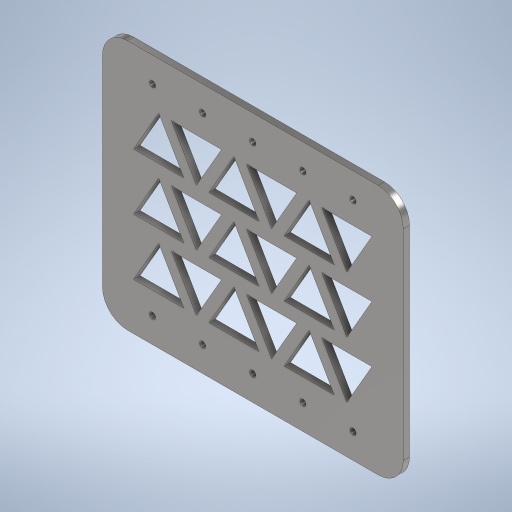
# Autodesk Inventor part: Low Frame to Mid Frame bracket
Saved by Autodesk Inventor 2023 (Build 270158030, 158C)
## iProperties
Created: 2022-07-20
Part Number: Low Frame to Mid Frame bracket
Material: Generic
Document SubType Name: Modeling
Designer: rm0990889
Density: 1 g/cm^3
Appearance: Semi-Polished
Author: rm0990889
Autodesk Inventor part; units mm, degrees
ref_plane "YZ Plane" through (0, 0, 0) normal (1, 0, 0) x (0, 1, 0)
ref_plane "XZ Plane" through (0, 0, 0) normal (0, 1, 0) x (-1, 0, 0)
ref_plane "XY Plane" through (0, 0, 0) normal (0, 0, 1) x (1, 0, 0)
sketch "Sketch1" plane through (0, 0, 0) normal (0, 0, 1) x (1, 0, 0)
  line L0 (0, 0) -> (152.4, 0)
  line L1 (152.4, 25.4) -> (152.4, 127)
  line L2 (152.4, 152.4) -> (0, 152.4)
  line L3 (0, 127) -> (0, 25.4)
  circle A0 centre (25.4, 127) radius 1.5875
  circle A1 centre (50.8, 127) radius 1.5875
  circle A2 centre (76.2, 127) radius 1.5875
  circle A3 centre (101.6, 127) radius 1.5875
  circle A4 centre (127, 127) radius 1.5875
  circle A5 centre (25.4, 25.4) radius 1.5875
  circle A6 centre (50.8, 25.4) radius 1.5875
  circle A7 centre (76.2, 25.4) radius 1.5875
  circle A8 centre (101.6, 25.4) radius 1.5875
  circle A9 centre (127, 25.4) radius 1.5875
  line L4 (41.275, 36.6265) -> (15.875, 36.6265)
  line L5 (15.875, 36.6265) -> (28.575, 58.6235)
  line L6 (28.575, 58.6235) -> (41.275, 36.6265)
  line L7 (60.325, 58.6235) -> (47.625, 36.6265)
  line L8 (47.625, 36.6265) -> (34.925, 58.6235)
  line L9 (34.925, 58.6235) -> (60.325, 58.6235)
  line L10 (98.425, 58.6235) -> (85.725, 36.6265)
  line L11 (73.025, 58.6235) -> (98.425, 58.6235)
  line L12 (85.725, 36.6265) -> (73.025, 58.6235)
  line L13 (66.675, 58.6235) -> (79.375, 36.6265)
  line L14 (53.975, 36.6265) -> (66.675, 58.6235)
  line L15 (79.375, 36.6265) -> (53.975, 36.6265)
  line L16 (136.525, 58.6235) -> (123.825, 36.6265)
  line L17 (111.125, 58.6235) -> (136.525, 58.6235)
  line L18 (123.825, 36.6265) -> (111.125, 58.6235)
  line L19 (104.775, 58.6235) -> (117.475, 36.6265)
  line L20 (92.075, 36.6265) -> (104.775, 58.6235)
  line L21 (117.475, 36.6265) -> (92.075, 36.6265)
  line L22 (0, 36.6265) -> (15.875, 36.6265)
  line L23 (136.525, 58.6235) -> (152.4, 58.6235)
  line L24 (104.775, 87.1985) -> (117.475, 65.2015)
  line L25 (123.825, 65.2015) -> (111.125, 87.1985)
  line L26 (136.525, 87.1985) -> (123.825, 65.2015)
  line L27 (111.125, 87.1985) -> (136.525, 87.1985)
  line L28 (117.475, 65.2015) -> (92.075, 65.2015)
  line L29 (41.275, 65.2015) -> (15.875, 65.2015)
  line L30 (15.875, 65.2015) -> (28.575, 87.1985)
  line L31 (28.575, 87.1985) -> (41.275, 65.2015)
  line L32 (60.325, 87.1985) -> (47.625, 65.2015)
  line L33 (47.625, 65.2015) -> (34.925, 87.1985)
  line L34 (34.925, 87.1985) -> (60.325, 87.1985)
  line L35 (92.075, 65.2015) -> (104.775, 87.1985)
  line L36 (73.025, 87.1985) -> (98.425, 87.1985)
  line L37 (85.725, 65.2015) -> (73.025, 87.1985)
  line L38 (66.675, 87.1985) -> (79.375, 65.2015)
  line L39 (53.975, 65.2015) -> (66.675, 87.1985)
  line L40 (79.375, 65.2015) -> (53.975, 65.2015)
  line L41 (98.425, 87.1985) -> (85.725, 65.2015)
  line L42 (104.775, 115.7735) -> (117.475, 93.7765)
  line L43 (123.825, 93.7765) -> (111.125, 115.7735)
  line L44 (136.525, 115.7735) -> (123.825, 93.7765)
  line L45 (111.125, 115.7735) -> (136.525, 115.7735)
  line L46 (117.475, 93.7765) -> (92.075, 93.7765)
  line L47 (41.275, 93.7765) -> (15.875, 93.7765)
  line L48 (15.875, 93.7765) -> (28.575, 115.7735)
  line L49 (28.575, 115.7735) -> (41.275, 93.7765)
  line L50 (60.325, 115.7735) -> (47.625, 93.7765)
  line L51 (47.625, 93.7765) -> (34.925, 115.7735)
  line L52 (34.925, 115.7735) -> (60.325, 115.7735)
  line L53 (92.075, 93.7765) -> (104.775, 115.7735)
  line L54 (73.025, 115.7735) -> (98.425, 115.7735)
  line L55 (85.725, 93.7765) -> (73.025, 115.7735)
  line L56 (66.675, 115.7735) -> (79.375, 93.7765)
  line L57 (53.975, 93.7765) -> (66.675, 115.7735)
  line L58 (79.375, 93.7765) -> (53.975, 93.7765)
  line L59 (98.425, 115.7735) -> (85.725, 93.7765)
  line L60 (15.875, 36.6265) -> (15.875, 0)
  line L61 (28.575, 115.7735) -> (28.575, 152.4)
  line L62 (12.7, 12.7) -> (139.7, 12.7)
  line L63 (12.7, 139.7) -> (139.7, 139.7)
  arc A10 (0, 25.4) -> (12.7, 12.7) centre (12.7, 25.4) ccw
  arc A11 (139.7, 12.7) -> (152.4, 25.4) centre (139.7, 25.4) ccw
  arc A12 (152.4, 127) -> (139.7, 139.7) centre (139.7, 127) ccw
  arc A13 (12.7, 139.7) -> (0, 127) centre (12.7, 127) ccw
  point P0 (28.575, 43.9588)
  point P1 (28.575, 36.6265)
  point P2 (47.625, 51.2912)
  point P3 (85.725, 51.2912)
  point P4 (66.675, 43.9588)
  point P5 (66.675, 36.6265)
  point P6 (123.825, 51.2912)
  point P7 (104.775, 43.9588)
  point P8 (104.775, 36.6265)
  point P9 (123.825, 79.8662)
  point P10 (104.775, 65.2015)
  point P11 (28.575, 72.5338)
  point P12 (28.575, 65.2015)
  point P13 (47.625, 79.8662)
  point P14 (104.775, 72.5338)
  point P15 (85.725, 79.8662)
  point P16 (66.675, 72.5338)
  point P17 (66.675, 65.2015)
  point P18 (123.825, 108.4412)
  point P19 (104.775, 93.7765)
  point P20 (28.575, 101.1088)
  point P21 (28.575, 93.7765)
  point P22 (47.625, 108.4412)
  point P23 (104.775, 101.1088)
  point P24 (85.725, 108.4412)
  point P25 (66.675, 101.1088)
  point P26 (66.675, 93.7765)
  dimension "d0" = 152.4
  dimension "d1" = 152.4
  dimension "d2" = 3.175
  dimension "d3" = 25.4
  dimension "d4" = 25.4
  dimension "d7" = 25.4
  dimension "d12" = 3.175
  dimension "d13" = 25.4
  dimension "d14" = 25.4
  dimension "d17" = 25.4
  dimension "d22" = 25.4
  dimension "d23" = 25.4
  dimension "d24" = 0
  dimension "d25" = 6.35
  dimension "d29" = 38.1
  dimension "d37" = 28.575
  dimension "d42" = 12.7
  dimension "d43" = 12.7
  dimension "d44" = 12.7
  constraints: 128 end point, 14 centre point, 8 point on circle, 8 point on line, 8 tangent, 6 horizontal, 5 perpendicular, 4 parallel, 3 equal radius, 2 vertical, 1 horizontal alignment, 1 midpoint, 150 other
  measures "d0" distance of L2.end L2.start
  measures "d1" distance of L2.start L0.end
  measures "d2" diameter of A0
  measures "d3" distance from line of L2 A0.centre
  measures "d4" distance from line of L3 A0.centre
  measures "d7" distance of A0.centre A1.centre
  measures "d12" diameter of A5
  measures "d13" distance from line of L3 A5.centre
  measures "d14" distance from line of L0 A5.centre
  measures "d17" distance of A5.centre A6.centre
  measures "d22" distance of L4.start L4.end
  measures "d23" distance of L8.end L7.start
  measures "d24" vertical distance of L7.end L4.start
  measures "d25" distance of L8.end L5.end
  measures "d29" distance of L7.end L10.end
  measures "d37" distance of L19.end L24.end
  measures "d42" distance from line of L63 A4.centre
  measures "d43" distance from line of L62 A9.centre
  measures "d44" radius of A10
extrude "Extrusion1" add sketch "Sketch1" along normal blind 3.175
body "Solid1"
